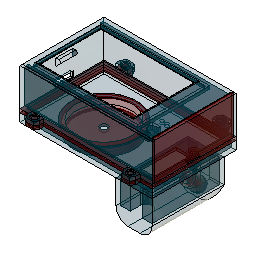
DicaPi v26 (Autodesk Fusion 360 design; units mm, degrees)
Autodesk Fusion 360 part; units mm, degrees
note: some values were not read from the file. Chosen so that the rebuilt part matches the saved one: which bodies a step acts on; which face or edge a step refers to. Set by a fixed rule: which sketch regions a step uses.
sketch "Mount-Grip" plane through (0, 0, 0) normal (0, 0, 1) x (1, 0, 0)
  line L0 (0, 0) -> (110, 0)
  line L1 (110, 0) -> (110, 70)
  line L2 (110, 70) -> (0, 70)
  line L3 (0, 70) -> (0, 0)
  circle A0 centre (35, 35) radius 25
  circle A1 centre (35, 35) radius 23
  line L4 (2, 68) -> (108, 68)
  line L5 (108, 68) -> (108, 2)
  line L6 (108, 2) -> (2, 2)
  line L7 (2, 2) -> (2, 68)
  circle A2 centre (60, 58.5) radius 1.5
  circle A3 centre (64, 58.5) radius 1.5
  line L8 (110, 60) -> (80, 60)
  line L9 (80, 60) -> (80, 0)
  line L10 (80, 0) -> (110, 0)
  line L11 (110, 0) -> (110, 60)
  circle A4 centre (95, 50) radius 2.5
  circle A5 centre (95, 10) radius 2.5
  line L12 (150, 60) -> (180, 60)
  line L13 (180, 60) -> (180, 0)
  line L14 (180, 0) -> (150, 0)
  line L15 (150, 0) -> (150, 60)
  line L16 (168, 51.7321) -> (165, 53.4641)
  line L17 (165, 53.4641) -> (162, 51.7321)
  line L18 (162, 51.7321) -> (162, 48.2679)
  line L19 (162, 48.2679) -> (165, 46.5359)
  line L20 (165, 46.5359) -> (168, 48.2679)
  line L21 (168, 48.2679) -> (168, 51.7321)
  line L22 (168, 11.7321) -> (165, 13.4641)
  line L23 (165, 13.4641) -> (162, 11.7321)
  line L24 (162, 11.7321) -> (162, 8.2679)
  line L25 (162, 8.2679) -> (165, 6.5359)
  line L26 (165, 6.5359) -> (168, 8.2679)
  line L27 (168, 8.2679) -> (168, 11.7321)
  circle A6 centre (35, 35) radius 27
  circle A7 centre (35, 35) radius 3
  circle A8 centre (165, 10) radius 2
  circle A9 centre (165, 50) radius 2
  line L28 (152, 15) -> (178, 15)
  line L29 (178, 15) -> (178, 45)
  line L30 (178, 45) -> (152, 45)
  line L31 (152, 45) -> (152, 15)
  line L32 (178, 15) -> (170, 15)
  line L33 (170, 15) -> (170, 2)
  line L34 (170, 2) -> (178, 2)
  line L35 (178, 2) -> (178, 15)
  line L36 (160, 15) -> (152, 15)
  line L37 (152, 15) -> (152, 2)
  line L38 (152, 2) -> (160, 2)
  line L39 (160, 2) -> (160, 15)
  line L40 (152, 45) -> (160, 45)
  line L41 (160, 45) -> (160, 58)
  line L42 (160, 58) -> (152, 58)
  line L43 (152, 58) -> (152, 45)
  line L44 (170, 58) -> (178, 58)
  line L45 (178, 58) -> (178, 45)
  line L46 (178, 45) -> (170, 45)
  line L47 (170, 45) -> (170, 58)
  line L48 (85, 15) -> (105, 15)
  line L49 (105, 15) -> (105, 45)
  line L50 (105, 45) -> (85, 45)
  line L51 (85, 45) -> (85, 15)
  point P0 (165, 50)
  point P1 (165, 10)
  dimension "d1" = 110
  dimension "d2" = 70
  dimension "d3" = 5
  dimension "d4" = 5
  dimension "d5" = 3
  dimension "d6" = 3
  dimension "d7" = 54
  dimension "d8" = 6
  dimension "d45" = 4
  dimension "d46" = 4
  constraint horizontal L0
  constraint vertical L1
  constraint horizontal L2
  constraint vertical L3
  constraint coincident L0.start L3.end
  constraint concentric A0 A1
  constraint horizontal L4
  constraint vertical L5
  constraint horizontal L6
  constraint vertical L7
  constraint horizontal L8
  constraint vertical L9
  constraint horizontal L10
  constraint vertical L11
  constraint coincident L0 L9.end
  constraint coincident L1 L8.start
  constraint horizontal L12
  constraint vertical L13
  constraint horizontal L14
  constraint vertical L15
  constraint concentric A1 A6
  constraint concentric A0 A7
  constraint coincident P1 A8.centre
  constraint coincident P0 A9.centre
  constraint horizontal L28
  constraint vertical L29
  constraint horizontal L30
  constraint vertical L31
  constraint horizontal L32
  constraint vertical L33
  constraint horizontal L34
  constraint vertical L35
  constraint horizontal L36
  constraint vertical L37
  constraint horizontal L38
  constraint vertical L39
  constraint coincident L28 L36.start
  constraint horizontal L40
  constraint vertical L41
  constraint horizontal L42
  constraint vertical L43
  constraint horizontal L44
  constraint vertical L45
  constraint horizontal L46
  constraint vertical L47
  constraint horizontal L48
  constraint vertical L49
  constraint horizontal L50
  constraint vertical L51
  measures "d1" distance of L0.start L0.end
  measures "d2" distance of L0.start L2.end
  measures "d3" diameter of A4
  measures "d4" diameter of A5
  measures "d5" distance of P0 L21
  measures "d6" distance of P1 L27
  measures "d7" diameter of A6
  measures "d8" diameter of A7
  measures "d45" diameter of A8
  measures "d46" diameter of A9
extrude "Extrude1" add sketch "Mount-Grip" along normal blind 2 contours L0 L1 L2 L3 L4 L5 L6 L7 L8 L9 | L0 L1 L5 L6 L8 L9 L10 L11 | L5 L6 L8 L9 | L4 L5 L6 L7 L8 L9 | A6 | L48 L49 L50 L51 makes body 1
extrude "Extrude2" add sketch "Mount-Grip" along normal blind 7 contours L0 L1 L2 L3 L4 L5 L6 L7 L8 L9 | L0 L1 L5 L6 L8 L9 L10 L11 bodies 1
chamfer "Chamfer1" distance 1 angle 45 1 edges at (92.6692, 50.904, 2) on bodies 1
chamfer "Chamfer2" distance 1 angle 45 1 edges at (92.6692, 10.904, 2) on bodies 1
extrude "Extrude3" add sketch "Mount-Grip" along normal blind 2 separate body contours A6 makes body 2
extrude "Extrude4" add sketch "Mount-Grip" along normal blind 2 contours A0 bodies 2
extrude "Extrude5" add sketch "Mount-Grip" against normal blind 2 contours A0 bodies 2
extrude "Extrude6" add sketch "Mount-Grip" along normal blind 2 contours A1 bodies 2
move_body "Move1" bodies 2 to x (1, 0, 0) y (0, 1, 0) z (0, 0, 1) at (0, 0, 2)
extrude "Extrude7" cut sketch "Mount-Grip" along normal blind 32 contours A1 bodies 2
extrude "Extrude8" add sketch "Mount-Grip" against normal blind 4 contours A0 bodies 2
extrude "Extrude9" add 1 faces at (59.2403, 33.758, -4) along direction (0, 0, -1) blind 2 on bodies 2 bodies 2
extrude "Extrude10" add sketch "Mount-Grip" against normal blind 4 contours A1 bodies 2
extrude "Extrude11" cut sketch "Mount-Grip" against normal blind 2 contours A1 bodies 2
extrude "Extrude12" cut sketch "Mount-Grip" along normal blind 4 contours A6 bodies 1
extrude "Extrude13" add sketch "Mount-Grip" along normal blind 1 contours A6 bodies 1
extrude "Extrude14" cut 1 faces at (60.4805, 32.516, 4) along direction (0, 0, -1) blind 1 on bodies 2 bodies 2
move_body "Move2" bodies 2 to x (1, 0, 0) y (0, 1, 0) z (0, 0, 1) at (0, 0, -1)
extrude "Extrude15" add sketch "Mount-Grip" along normal blind 30 separate body contours L12 L13 L14 L15 | L16 L17 L18 L19 L20 L21 | L22 L23 L24 L25 L26 L27 | A8 | A9 | L28 L29 L30 L31 L32 L36 L40 L46 | L28 L36 L37 L38 L39 | L30 L40 L41 L42 L43 | L28 L32 L33 L34 L35 | L30 L44 L45 L46 L47 makes body 3
chamfer "Chamfer3" distance 10 angle 45 1 edges at (165, 60, 30) on bodies 3
fillet "Fillet1" radius 10 2 edges at (180, 25, 30) (150, 25, 30) on bodies 3
extrude "Extrude16" cut sketch "Mount-Grip" along normal blind 3 contours L16 L17 L18 L19 L20 L21 | L22 L23 L24 L25 L26 L27 | A8 | A9 bodies 3
extrude "Extrude17" cut sketch "Mount-Grip" along normal blind 15 contours A8 | A9 bodies 3
extrude "Extrude18" cut sketch "Mount-Grip" along normal blind 20 contours L28 L29 L30 L31 L32 L36 L40 L46 | L28 L36 L37 L38 L39 | L30 L40 L41 L42 L43 | L28 L32 L33 L34 L35 | L30 L44 L45 L46 L47 bodies 3
fillet "Fillet2" radius 5 4 edges at (170, 15, 10) (160, 15, 10) (170, 45, 10) (160, 45, 10) on bodies 3
sketch "Button" plane through (0, 40, 40) normal (0, 0.707107, 0.707107) x (-1, 0, 0)
  ellipse E0 centre (-160, -28.2843) end of major axis (-160, -14.1421) minor radius 10 (-150, -28.2843) -> (-160, -14.1421) ccw
  line L0 (-160, -14.1421) -> (-170, -14.1421)
  ellipse E1 centre (-170, -28.2843) end of major axis (-170, -14.1421) minor radius 10 (-170, -14.1421) -> (-180, -28.2843) ccw
  line L1 (-180, -28.2843) -> (-150, -28.2843)
  line L2 (-161.5, -24.5) -> (-168.5, -24.5)
  line L3 (-168.5, -24.5) -> (-168.5, -17.5)
  line L4 (-168.5, -17.5) -> (-161.5, -17.5)
  line L5 (-161.5, -17.5) -> (-161.5, -24.5)
  line L6 (-161.5, -24.5) -> (-168.5, -17.5) construction
  line L7 (-168.5, -24.5) -> (-161.5, -17.5) construction
  circle A0 centre (-165, -21) radius 5
  circle A1 centre (-165, -21) radius 5.5
  circle A2 centre (-165, -21) radius 1.5
  point P0 (-165, -21)
  dimension "d52" = 7
  dimension "d53" = 7
  dimension "d68" = 3
  constraint horizontal L2
  constraint perpendicular L2 L3
  constraint parallel L2 L4
  constraint parallel L3 L5
  constraint coincident L6 P0
  constraint coincident L7 P0
  constraint coincident P0 A0.centre
  constraint concentric A0 A1
  constraint concentric A1 A2
  measures "d52" distance of L3.end L4.end
  measures "d53" distance of L2.end L3.end
  measures "d68" diameter of A2
extrude "Extrude19" cut sketch "Button" against normal blind 89 contours L2 L3 L4 L5 | A2 bodies 3
extrude "Extrude20" cut sketch "Button" against normal blind 43.5 contours A0 bodies 3
extrude "Extrude21" cut sketch "Button" against normal blind 57.5 contours A1 bodies 3
extrude "Extrude22" add sketch "Button" against normal blind 2 contours A1 bodies 3
extrude "Extrude23" add sketch "Button" against normal blind 1 separate body contours A1 makes body 4
extrude "Extrude24" add sketch "Button" against normal blind 1 contours L2 L3 L4 L5 | A0 | A2 bodies 4
extrude "Extrude25" add sketch "Button" along normal blind 3 contours L2 L3 L4 L5 | A0 | A2 bodies 4
extrude "Extrude26" cut sketch "Button" against normal blind 9 contours A2 bodies 4
move_body "Move3" bodies 4 to x (1, 0, 0) y (0, 1, 0) z (0, 0, 1) at (0, -2, -2)
move_body "Move4" bodies 4 to x (1, 0, 0) y (0, 1, 0) z (0, 0, 1) at (0, 0.5, 0.5)
fillet "Fillet3" radius 1 1 edges at (169.6616, 56.7491, 24.4936) on bodies 4
extrude "Extrude27" cut sketch "Mount-Grip" along normal blind 26 contours L48 L49 L50 L51 bodies 1
move_body "Move5" bodies 3 4 to x (-1, 0, 0) y (0, 1, 0) z (0, 0, -1) at (260, 0, 0)
extrude "Extrude28" add sketch "Button" against normal blind 10 separate body contours L2 L3 L4 L5 | A0 makes body 5
extrude "Extrude29" cut sketch "Button" against normal blind 4 contours L2 L3 L4 L5 bodies 5
move_face "OffsetFaces1" offset -2 1 faces at (164.7395, 48.1478, 20.5384) on bodies 5
extrude "Extrude30" add sketch "Button" against normal blind 10 contours A1 bodies 5
move_body "Move6" bodies 5 to x (-1, 0, 0) y (0, 1, 0) z (0, 0, -1) at (260, -2.88, 2.8812)
sketch "BodyBase" plane through (0, 0, 0) normal (0, 0, 1) x (1, 0, 0)
  line L0 (0, 0) -> (110, 0)
  line L1 (110, 0) -> (110, 70)
  line L2 (110, 70) -> (0, 70)
  line L3 (0, 70) -> (0, 0)
  line L4 (85, 35) -> (85, 60.5)
  line L5 (85, 60.5) -> (7, 60.5)
  line L6 (7, 60.5) -> (7, 35)
  line L7 (85, 35) -> (85, 9.5)
  line L8 (85, 9.5) -> (7, 9.5)
  line L9 (7, 9.5) -> (7, 35)
  line L10 (91, 35) -> (91, 63)
  line L11 (91, 63) -> (4, 63)
  line L12 (4, 63) -> (4, 35)
  line L13 (91, 35) -> (91, 7)
  line L14 (91, 7) -> (4, 7)
  line L15 (4, 7) -> (4, 35)
  line L16 (2, 68) -> (108, 68)
  line L17 (108, 68) -> (108, 2)
  line L18 (108, 2) -> (2, 2)
  line L19 (2, 2) -> (2, 68)
  line L20 (110, 68) -> (95, 68)
  line L21 (95, 68) -> (95, 2)
  line L22 (95, 2) -> (110, 2)
  line L23 (110, 2) -> (110, 68)
  line L24 (110, 68) -> (106, 68)
  line L25 (106, 68) -> (106, 2)
  line L26 (106, 2) -> (110, 2)
  line L27 (110, 2) -> (110, 68)
  line L28 (3, 67) -> (107, 67)
  line L29 (107, 67) -> (107, 3)
  line L30 (107, 3) -> (3, 3)
  line L31 (3, 3) -> (3, 67)
  dimension "d84" = 78
  dimension "d85" = 25.5
  dimension "d86" = 25.5
  dimension "d87" = 28
  constraint horizontal L0
  constraint vertical L1
  constraint horizontal L2
  constraint vertical L3
  constraint coincident L0.start L3.end
  constraint vertical L4
  constraint horizontal L5
  constraint vertical L6
  constraint vertical L7
  constraint horizontal L8
  constraint vertical L9
  constraint vertical L10
  constraint horizontal L11
  constraint vertical L12
  constraint vertical L13
  constraint horizontal L14
  constraint vertical L15
  constraint horizontal L16
  constraint vertical L17
  constraint horizontal L18
  constraint vertical L19
  constraint horizontal L20
  constraint vertical L21
  constraint horizontal L22
  constraint vertical L23
  constraint coincident L18 L21.end
  constraint coincident L1 L20.start
  constraint horizontal L24
  constraint vertical L25
  constraint horizontal L26
  constraint vertical L27
  constraint coincident L22 L25.end
  constraint horizontal L28
  constraint vertical L29
  constraint horizontal L30
  constraint vertical L31
  measures "d84" distance of L6.end L4.start
  measures "d85" distance of L6.end L5.end
  measures "d86" distance of L6.end L8.end
  measures "d87" distance of L12.end L14.end
extrude "Extrude31" add sketch "BodyBase" along normal blind 35 separate body contours L0 L1 L2 L3 L16 L18 L19 L20 L22 L24 L26 | L1 L17 L20 L22 L23 L24 L26 L27 | L16 L17 L18 L20 L22 L24 L25 L26 L28 L29 L30 | L18 L21 L22 L25 L30 | L16 L20 L21 L25 L28 | L16 L18 L19 L21 L28 L30 L31 | L21 L25 L28 L30 | L25 L28 L29 L30 | L21 L28 L30 L31 | L4 L5 L6 L7 L8 L9 | L10 L11 L12 L13 L14 L15 makes body 6
sketch "Face" plane through (0, 0, 35) normal (0, 0, 1) x (-1, 0, 0)
  line L0 (-110, 0) -> (-110, -70)
  line L1 (-110, -70) -> (0, -70)
  line L2 (0, -70) -> (0, 0)
  line L3 (0, 0) -> (-110, 0)
  line L4 (-95, -68) -> (-110, -68)
  line L5 (-110, -68) -> (-110, -2)
  line L6 (-110, -2) -> (-95, -2)
  line L7 (-95, -2) -> (-95, -68)
  line L8 (-108, -68) -> (-110, -68)
  line L9 (-110, -68) -> (-110, -2)
  line L10 (-110, -2) -> (-108, -2)
  line L11 (-108, -2) -> (-108, -68)
  line L12 (-108, -2) -> (-106, -2)
  line L13 (-106, -2) -> (-106, -68)
  line L14 (-106, -68) -> (-108, -68)
  line L15 (-108, -68) -> (-108, -2)
  line L16 (-7, -9.5) -> (-85, -9.5)
  line L17 (-85, -9.5) -> (-85, -60.5)
  line L18 (-85, -60.5) -> (-7, -60.5)
  line L19 (-7, -60.5) -> (-7, -9.5)
  line L20 (-4, -63) -> (-91, -63)
  line L21 (-91, -63) -> (-91, -7)
  line L22 (-91, -7) -> (-4, -7)
  line L23 (-4, -7) -> (-4, -63)
  line L24 (-2, -65) -> (-93, -65)
  line L25 (-93, -65) -> (-93, -5)
  line L26 (-93, -5) -> (-2, -5)
  line L27 (-2, -5) -> (-2, -65)
  constraint horizontal L4
  constraint vertical L5
  constraint horizontal L6
  constraint vertical L7
  constraint coincident L0 L5.end
  constraint horizontal L8
  constraint vertical L9
  constraint horizontal L10
  constraint vertical L11
  constraint coincident L4 L8.start
  constraint horizontal L12
  constraint vertical L13
  constraint horizontal L14
  constraint vertical L15
  constraint coincident L4 L13.end
  constraint horizontal L16
  constraint vertical L17
  constraint horizontal L18
  constraint vertical L19
  constraint horizontal L20
  constraint vertical L21
  constraint horizontal L22
  constraint vertical L23
  constraint horizontal L24
  constraint vertical L25
  constraint horizontal L26
  constraint vertical L27
sketch "Adhesive" plane through (0, 0, 0) normal (0, 0, -1) x (1, 0, 0)
  line L0 (110, -70) -> (110, 0)
  line L1 (110, 0) -> (0, 0)
  line L2 (0, 0) -> (0, -70)
  line L3 (0, -70) -> (110, -70)
  line L4 (2, -2) -> (106, -2)
  line L5 (106, -2) -> (106, -68)
  line L6 (106, -68) -> (2, -68)
  line L7 (2, -68) -> (2, -2)
  line L8 (108, -2) -> (110, -2)
  line L9 (110, -2) -> (110, -68)
  line L10 (110, -68) -> (108, -68)
  line L11 (108, -68) -> (108, -2)
  line L12 (3, -3) -> (107, -3)
  line L13 (107, -3) -> (107, -67)
  line L14 (107, -67) -> (3, -67)
  line L15 (3, -67) -> (3, -3)
  line L16 (108, -2) -> (106, -2)
  line L17 (106, -2) -> (106, -68)
  line L18 (106, -68) -> (108, -68)
  line L19 (108, -68) -> (108, -2)
  constraint horizontal L4
  constraint vertical L5
  constraint horizontal L6
  constraint vertical L7
  constraint horizontal L8
  constraint vertical L9
  constraint horizontal L10
  constraint vertical L11
  constraint coincident L0 L9.end
  constraint horizontal L12
  constraint vertical L13
  constraint horizontal L14
  constraint vertical L15
  constraint horizontal L16
  constraint vertical L17
  constraint horizontal L18
  constraint vertical L19
extrude "Extrude32" cut sketch "Adhesive" against normal blind 33.5 contours L5 L11 L12 L13 L14 L16 L17 L18 L19 | L4 L5 L6 L7 L12 L14 L15 L17 | L5 L12 L14 L15 L17 | L5 L12 L13 L14 L17 bodies 6
extrude "Extrude33" add sketch "Adhesive" against normal blind 2 contours L5 L11 L12 L13 L14 L16 L17 L18 L19 | L4 L5 L6 L7 L12 L14 L15 L17 bodies 6
extrude "Extrude34" add sketch "Adhesive" along normal blind 2 contours L5 L11 L12 L13 L14 L16 L17 L18 L19 | L4 L5 L6 L7 L12 L14 L15 L17 bodies 6
extrude "Extrude35" cut sketch "Face" against normal blind 5 contours L16 L17 L18 L19 bodies 6
extrude "Extrude36" add sketch "Face" against normal blind 4 contours L24 L25 L26 L27 bodies 6
extrude "Extrude37" cut sketch "Face" against normal blind 2 contours L0 L4 L5 L6 L8 L9 L10 L11 L15 | L4 L6 L11 L12 L13 L14 L15 | L4 L6 L7 L13 bodies 6
extrude "Extrude38" cut sketch "Face" against normal blind 30 contours L0 L4 L5 L6 L8 L9 L10 L11 L15 bodies 6
extrude "Extrude39" add sketch "Face" against normal blind 1.5 contours L4 L6 L7 L13 bodies 6
extrude "Extrude40" add 1 faces at (106, 24, 34.5) along direction (1, 0, 0) blind 2 on bodies 6 bodies 6
chamfer "Chamfer4" distance 1 angle 45 1 edges at (108, 35, 33.5) on bodies 6
sketch "IOCap" plane through (110, 0, 0) normal (1, 0, 0) x (0, 1, 0)
  line L0 (2, 5) -> (2, 35)
  line L1 (2, 35) -> (0, 35)
  line L2 (0, 35) -> (0, 0)
  line L3 (0, 0) -> (70, 0)
  line L4 (70, 0) -> (70, 35)
  line L5 (70, 35) -> (68, 35)
  line L6 (68, 35) -> (68, 5)
  line L7 (68, 5) -> (2, 5)
  line L8 (2, 35) -> (68, 35)
  line L9 (68, 35) -> (68, 3)
  line L10 (68, 3) -> (2, 3)
  line L11 (2, 3) -> (2, 35)
  line L12 (30, 3) -> (40, 3)
  line L13 (40, 3) -> (40, 4)
  line L14 (40, 4) -> (30, 4)
  line L15 (30, 4) -> (30, 3)
  line L16 (30, 3) -> (40, 3)
  line L17 (40, 3) -> (40, 5)
  line L18 (40, 5) -> (30, 5)
  line L19 (30, 5) -> (30, 3)
  constraint horizontal L8
  constraint vertical L9
  constraint horizontal L10
  constraint vertical L11
  constraint coincident L0.end L1.start
  constraint horizontal L12
  constraint vertical L13
  constraint horizontal L14
  constraint vertical L15
  constraint coincident L10 L12.start
  constraint horizontal L16
  constraint vertical L17
  constraint horizontal L18
  constraint vertical L19
  constraint coincident L7 L17.end
extrude "Extrude41" add 1 faces at (108, 46, 3) along direction (-1, 0, 0) blind 1 on bodies 6 bodies 6
extrude "Extrude42" cut sketch "IOCap" against normal blind 2 contours L7 L10 L11 L15 L19 | L7 L14 L17 L18 L19 | L7 L9 L10 L13 L17 | L10 L12 L13 L14 L15 L16 L17 L19 bodies 6
extrude "Extrude43" add sketch "IOCap" against normal blind 2 separate body contours L0 L6 L7 L8 L9 L11 L18 | L7 L10 L11 L15 L19 | L7 L9 L10 L13 L17 makes body 7
extrude "Extrude44" add sketch "IOCap" against normal blind 1 contours L7 L14 L17 L18 L19 bodies 7
sketch "Body-Top" plane through (0, 70, 0) normal (0, 1, 0) x (-1, 0, 0)
  line L0 (-110, 0) -> (0, 0)
  line L1 (0, 0) -> (0, 35)
  line L2 (0, 35) -> (-110, 35)
  line L3 (-110, 35) -> (-110, 0)
  line L4 (-100, 0) -> (-90, 0)
  line L5 (-90, 0) -> (-90, 5)
  line L6 (-90, 5) -> (-100, 5)
  line L7 (-100, 5) -> (-100, 0)
  line L8 (-10, 0) -> (-20, 0)
  line L9 (-20, 0) -> (-20, 5)
  line L10 (-20, 5) -> (-10, 5)
  line L11 (-10, 5) -> (-10, 0)
  line L12 (-20, 33) -> (-50, 33)
  line L13 (-50, 33) -> (-50, 18)
  line L14 (-50, 18) -> (-20, 18)
  line L15 (-20, 18) -> (-20, 33)
  line L16 (-23, 18) -> (-47, 18)
  line L17 (-47, 18) -> (-47, 33)
  line L18 (-47, 33) -> (-23, 33)
  line L19 (-23, 33) -> (-23, 18)
  constraint horizontal L4
  constraint vertical L5
  constraint horizontal L6
  constraint vertical L7
  constraint coincident L0 L4.start
  constraint horizontal L8
  constraint vertical L9
  constraint horizontal L10
  constraint vertical L11
  constraint coincident L0 L8.start
  constraint horizontal L12
  constraint vertical L13
  constraint horizontal L14
  constraint vertical L15
  constraint horizontal L16
  constraint vertical L17
  constraint horizontal L18
  constraint vertical L19
  constraint coincident L12 L17.end
  constraint coincident L14 L16.start
extrude "Extrude45" add sketch "Body-Top" along normal blind 15 separate body contours L12 L14 L16 L17 L18 L19 makes body 8
sketch "Body-Bottom" plane through (0, 0, 0) normal (0, -1, 0) x (1, 0, 0)
  line L0 (0, 0) -> (110, 0)
  line L1 (110, 0) -> (110, 35)
  line L2 (110, 35) -> (0, 35)
  line L3 (0, 35) -> (0, 0)
  line L4 (10, 0) -> (20, 0)
  line L5 (20, 0) -> (20, 5)
  line L6 (20, 5) -> (10, 5)
  line L7 (10, 5) -> (10, 0)
  line L8 (90, 0) -> (100, 0)
  line L9 (100, 0) -> (100, 5)
  line L10 (100, 5) -> (90, 5)
  line L11 (90, 5) -> (90, 0)
  constraint horizontal L4
  constraint vertical L5
  constraint horizontal L6
  constraint vertical L7
  constraint coincident L0 L4.start
  constraint horizontal L8
  constraint vertical L9
  constraint horizontal L10
  constraint vertical L11
  constraint coincident L0 L8.start
sketch "View-Guide" plane through (0, 0, 33) normal (0, 0, 1) x (-1, 0, 0)
  line L0 (-23, -70) -> (-47, -70)
  line L1 (-47, -70) -> (-47, -85)
  line L2 (-47, -85) -> (-23, -85)
  line L3 (-23, -85) -> (-23, -70)
  line L4 (-26, -83) -> (-44, -83)
  line L5 (-44, -83) -> (-44, -72)
  line L6 (-44, -72) -> (-26, -72)
  line L7 (-26, -72) -> (-26, -83)
  circle A0 centre (-35, -77.5) radius 5
  circle A1 centre (-35, -77.5) radius 4.75
  line L8 (-44, -77.25) -> (-26, -77.25)
  line L9 (-26, -77.25) -> (-26, -77.75)
  line L10 (-26, -77.75) -> (-44, -77.75)
  line L11 (-44, -77.75) -> (-44, -77.25)
  line L12 (-44, -77.25) -> (-26, -77.75) construction
  line L13 (-26, -77.25) -> (-44, -77.75) construction
  line L14 (-35.25, -72) -> (-34.75, -72)
  line L15 (-34.75, -72) -> (-34.75, -83)
  line L16 (-34.75, -83) -> (-35.25, -83)
  line L17 (-35.25, -83) -> (-35.25, -72)
  line L18 (-35.25, -72) -> (-34.75, -83) construction
  line L19 (-34.75, -72) -> (-35.25, -83) construction
  point P0 (-35, -77.5)
  point P1 (-35, -77.5)
  dimension "d119" = 18
  dimension "d120" = 11
  dimension "d123" = 9.5
  dimension "d124" = 0.5
  dimension "d125" = 0.5
  dimension "d126" = 11
  constraint horizontal L4
  constraint vertical L5
  constraint horizontal L6
  constraint vertical L7
  constraint concentric A0 A1
  constraint horizontal L8
  constraint perpendicular L8 L9
  constraint parallel L8 L10
  constraint parallel L9 L11
  constraint coincident L12 P1
  constraint coincident L13 P1
  constraint coincident P1 P0
  constraint horizontal L14
  constraint perpendicular L14 L15
  constraint parallel L14 L16
  constraint parallel L15 L17
  constraint coincident L18 P1
  constraint coincident L19 P1
  measures "d119" distance of L4.start L4.end
  measures "d120" distance of L4.start L6.end
  measures "d123" diameter of A1
  measures "d124" distance of L8.end L9.end
  measures "d125" distance of L15.end L16.end
  measures "d126" distance of L14.end L15.end
extrude "Extrude46" cut sketch "View-Guide" against normal blind 32 contours L4 L7 A0 L10 L15 | L4 A0 L15 L16 L17 | L7 A0 L8 L9 L10 | L4 L5 A0 L10 L17 | A0 A1 L10 L15 | A0 A1 L15 L17 | L6 L7 A0 L8 L15 | A0 A1 L8 L10 | A0 A1 L10 L17 | A1 L10 L15 | A1 L10 L15 L17 | A0 A1 L8 L15 | A1 L8 L10 L15 | L5 A0 L8 L10 L11 | A0 A1 L8 L10 | A1 L10 L17 | L8 L10 L15 L17 | L6 A0 L14 L15 L17 | A0 A1 L15 L17 | A1 L8 L15 | L5 L6 A0 L8 L17 | A0 A1 L8 L17 | A1 L8 L10 L17 | A1 L8 L15 L17 | A1 L8 L17 bodies 8
extrude "Extrude47" add sketch "View-Guide" against normal blind 0.5 contours L4 A0 L15 L16 L17 | L7 A0 L8 L9 L10 | A0 A1 L10 L15 | A0 A1 L15 L17 | A0 A1 L8 L10 | A0 A1 L10 L17 | A0 A1 L8 L15 | L5 A0 L8 L10 L11 | L6 A0 L14 L15 L17 | A0 A1 L15 L17 | A0 A1 L8 L17 picked at (-30.1719, -77.2778) bodies 8
extrude "Extrude48" add sketch "View-Guide" against normal blind 0.5 contours A0 A1 L8 L10 picked at (-39.8288, -77.6945) bodies 8
move_body "Move7" bodies 8 to x (-1, 0, 0) y (0, 1, 0) z (0, 0, -1) at (70, 0, 51)
extrude "Extrude49" add sketch "Body-Bottom" along normal blind 7 contours L0 L4 L5 L6 L7 | L0 L8 L9 L10 L11 bodies 6
extrude "Extrude50" add sketch "Body-Top" along normal blind 7 contours L0 L4 L5 L6 L7 | L0 L8 L9 L10 L11 bodies 6
chamfer "Chamfer5" distance 3 angle 45 8 edges at (10, 77, 2.5) (20, 77, 2.5) (90, 77, 2.5) (100, 77, 2.5) (10, -7, 2.5) (20, -7, 2.5) (100, -7, 2.5) (90, -7, 2.5) on bodies 6
sketch "Sketch14" plane through (0, 0, 0) normal (0, 0, -1) x (1, 0, 0)
  line L0 (93, 7) -> (90, 4)
  line L1 (90, 4) -> (90, 0)
  line L2 (90, 0) -> (20, 0)
  line L3 (20, 0) -> (20, 4)
  line L4 (20, 4) -> (17, 7)
  line L5 (17, 7) -> (13, 7)
  line L6 (13, 7) -> (10, 4)
  line L7 (10, 4) -> (10, 0)
  line L8 (10, 0) -> (0, 0)
  line L9 (0, 0) -> (0, -70)
  line L10 (0, -70) -> (10, -70)
  line L11 (10, -70) -> (10, -74)
  line L12 (10, -74) -> (13, -77)
  line L13 (13, -77) -> (17, -77)
  line L14 (17, -77) -> (20, -74)
  line L15 (20, -74) -> (20, -70)
  line L16 (20, -70) -> (90, -70)
  line L17 (90, -70) -> (90, -74)
  line L18 (90, -74) -> (93, -77)
  line L19 (93, -77) -> (97, -77)
  line L20 (97, -77) -> (100, -74)
  line L21 (100, -74) -> (100, -70)
  line L22 (100, -70) -> (110, -70)
  line L23 (110, -70) -> (110, 0)
  line L24 (110, 0) -> (100, 0)
  line L25 (100, 0) -> (100, 4)
  line L26 (100, 4) -> (97, 7)
  line L27 (97, 7) -> (93, 7)
  line L28 (2, -68) -> (2, -2)
  line L29 (2, -2) -> (108, -2)
  line L30 (108, -2) -> (108, -68)
  line L31 (108, -68) -> (2, -68)
  line L32 (13.2679, 6) -> (11.5359, 3)
  line L33 (11.5359, 3) -> (13.2679, 0)
  line L34 (13.2679, 0) -> (16.7321, 0)
  line L35 (16.7321, 0) -> (18.4641, 3)
  line L36 (18.4641, 3) -> (16.7321, 6)
  line L37 (16.7321, 6) -> (13.2679, 6)
  line L38 (93.268, 6) -> (91.5359, 3)
  line L39 (91.5359, 3) -> (93.268, 0)
  line L40 (93.268, 0) -> (96.7321, 0)
  line L41 (96.7321, 0) -> (98.4641, 3)
  line L42 (98.4641, 3) -> (96.7321, 6)
  line L43 (96.7321, 6) -> (93.268, 6)
  line L44 (13.2679, -70) -> (11.5359, -73)
  line L45 (11.5359, -73) -> (13.2679, -76)
  line L46 (13.2679, -76) -> (16.7321, -76)
  line L47 (16.7321, -76) -> (18.4641, -73)
  line L48 (18.4641, -73) -> (16.7321, -70)
  line L49 (16.7321, -70) -> (13.2679, -70)
  line L50 (93.268, -70) -> (91.5359, -73)
  line L51 (91.5359, -73) -> (93.268, -76)
  line L52 (93.268, -76) -> (96.7321, -76)
  line L53 (96.7321, -76) -> (98.4641, -73)
  line L54 (98.4641, -73) -> (96.7321, -70)
  line L55 (96.7321, -70) -> (93.268, -70)
  point P0 (15, 3)
  point P1 (95, 3)
  point P2 (15, -73)
  point P3 (95, -73)
delete_face "DeleteFace1" 1 faces at (98, -6, 1.6667) on bodies 6
delete_face "DeleteFace2" 1 faces at (12, -6, 3.3333) on bodies 6
delete_face "DeleteFace3" 1 faces at (92, -6, 3.3333) on bodies 6
delete_face "DeleteFace4" 1 faces at (19, -5, 1.6667) on bodies 6
delete_face "DeleteFace5" 1 faces at (98, 76, 3.3333) on bodies 6
delete_face "DeleteFace6" 1 faces at (91, 75, 1.6667) on bodies 6
delete_face "DeleteFace7" 1 faces at (19, 75, 1.6667) on bodies 6
delete_face "DeleteFace8" 1 faces at (12, 76, 3.3333) on bodies 6
chamfer "Chamfer6" distance 2 angle 60 8 edges at (10, -7, 2.5) (20, -7, 2.5) (90, -7, 2.5) (100, -7, 2.5) (20, 77, 2.5) (10, 77, 2.5) (90, 77, 2.5) (100, 77, 2.5) measured on face at (13.3333, -7, 1.6667) measured on face at (13.3333, -7, 1.6667) measured on face at (93.3333, -7, 1.6667) measured on face at (93.3333, -7, 1.6667) measured on face at (16.6667, 77, 1.6667) measured on face at (16.6667, 77, 1.6667) measured on face at (96.6667, 77, 1.6667) measured on face at (96.6667, 77, 1.6667) on bodies 6
extrude "Extrude51" add 1 faces at (37.3333, 67.6667, 2) along direction (0, 0, 1) blind 3 on bodies 6 bodies 6
extrude "Extrude52" add 4 faces at (94, -4.6906, 5) (16, -4.6906, 5) (16, 74.6906, 5) (94, 74.6906, 5) along direction (0, 0, 1) blind 1 on bodies 6 bodies 6
extrude "Extrude53" cut sketch "Sketch14" against normal blind 2 contours L32 L33 L34 L35 L36 L37 | L38 L39 L40 L41 L42 L43 | L44 L45 L46 L47 L48 L49 | L50 L51 L52 L53 L54 L55 bodies 6
sketch "Sketch15" plane through (0, 0, 6) normal (0, 0, 1) x (-1, 0, 0)
  line L0 (-100, -73.5359) -> (-98, -77)
  line L1 (-98, -77) -> (-92, -77)
  line L2 (-92, -77) -> (-90, -73.5359)
  line L3 (-90, -73.5359) -> (-90, -70)
  line L4 (-90, -70) -> (-100, -70)
  line L5 (-100, -70) -> (-100, -73.5359)
  circle A0 centre (-15, -73) radius 2
  circle A1 centre (-95, -73) radius 2
  circle A2 centre (-95, 3) radius 2
  circle A3 centre (-15, 3) radius 2
  circle A4 centre (-15, 3) radius 3
  circle A5 centre (-95, 3) radius 3
  circle A6 centre (-95, -73) radius 3
  circle A7 centre (-15, -73) radius 3
  constraint concentric A3 A4
  constraint concentric A2 A5
  constraint concentric A1 A6
  constraint concentric A0 A7
extrude "Extrude54" cut sketch "Sketch15" against normal blind 10 contours A0 | A1 | A2 | A3 bodies 6
extrude "Extrude55" cut sketch "Sketch15" against normal blind 1 contours A6 | A4 | A5 | A7 bodies 6
extrude "Extrude56" add 4 faces at (92.6673, 71.7107, 2) (15.0498, 75.6648, 2) (12.6673, -4.2893, 2) (97.3327, -4.2893, 2) along direction (0, 0, -1) blind 1 on bodies 6 bodies 6
split "Split1" by plane through (110, 40, 3) normal (0, 0, 1) bodies 6 makes body 9 at (100.3333, 43.5, 35)
sketch "Sketch17" plane through (0, 0, 0) normal (-1, 0, 0) x (0, -1, 0)
  line L0 (-70, 3) -> (0, 3)
  line L1 (0, 3) -> (0, 35)
  line L2 (0, 35) -> (-70, 35)
  line L3 (-70, 35) -> (-70, 3)
  line L4 (-35, 33.5) -> (-28, 33.5)
  line L5 (-28, 33.5) -> (-28, 9.5)
  line L6 (-28, 9.5) -> (-35, 9.5)
  line L7 (-35, 9.5) -> (-35, 33.5)
  line L8 (-35, 33.5) -> (-42, 33.5)
  line L9 (-42, 33.5) -> (-42, 9.5)
  line L10 (-42, 9.5) -> (-35, 9.5)
  line L11 (-35, 9.5) -> (-35, 33.5)
  line L12 (-42, 9.5) -> (-28, 9.5)
  line L13 (-28, 9.5) -> (-28, 5.5)
  line L14 (-28, 5.5) -> (-42, 5.5)
  line L15 (-42, 5.5) -> (-42, 9.5)
  line L16 (-5, 33.5) -> (-65, 33.5)
  line L17 (-65, 33.5) -> (-65, 26.5)
  line L18 (-65, 26.5) -> (-5, 26.5)
  line L19 (-5, 26.5) -> (-5, 33.5)
  line L20 (-65, 26.5) -> (-5, 26.5)
  line L21 (-5, 26.5) -> (-5, 25)
  line L22 (-5, 25) -> (-65, 25)
  line L23 (-65, 25) -> (-65, 26.5)
  line L24 (-42, 26.5) -> (-28, 26.5)
  line L25 (-28, 26.5) -> (-28, 21.5)
  line L26 (-28, 21.5) -> (-42, 21.5)
  line L27 (-42, 21.5) -> (-42, 26.5)
  dimension "d150" = 7
  dimension "d151" = 24
  dimension "d152" = 24
  dimension "d153" = 4
  dimension "d156" = 60
  dimension "d157" = 7
  constraint horizontal L4
  constraint vertical L5
  constraint horizontal L6
  constraint vertical L7
  constraint horizontal L8
  constraint vertical L9
  constraint horizontal L10
  constraint vertical L11
  constraint horizontal L12
  constraint vertical L13
  constraint horizontal L14
  constraint vertical L15
  constraint horizontal L16
  constraint vertical L17
  constraint horizontal L18
  constraint vertical L19
  constraint horizontal L20
  constraint vertical L21
  constraint horizontal L22
  constraint vertical L23
  constraint horizontal L24
  constraint vertical L25
  constraint horizontal L26
  constraint vertical L27
  constraint midpoint L5 L25.end
  constraint coincident L18 L24.start
  constraint coincident L9 L24.start
  measures "d150" distance of L4.start L4.end
  measures "d151" distance of L4.start L6.end
  measures "d152" distance of L4.start L6.end
  measures "d153" distance of L9.end L14.end
  measures "d156" distance of L16.start L16.end
  measures "d157" distance of L16.start L18.end
extrude "Extrude58" add sketch "Sketch17" against normal blind 7 contours L5 L7 L11 L18 L20 L22 L24 L25 | L7 L9 L11 L18 L20 L22 L24 L27 | L5 L7 L11 L22 L25 L26 | L7 L9 L11 L22 L26 L27 bodies 9
extrude "Extrude57" cut sketch "Sketch17" against normal blind 41 contours L6 L10 L12 L13 L14 L15 bodies 9
chamfer "Chamfer7" distance 4 angle 45 1 edges at (7, 35, 21.5) measured on face at (7, 37.3333, 24.8333) on bodies 9
fillet "Fillet4" radius 1 2 edges at (7, 35, 26.5) (7, 35, 25.5) on bodies 9
delete_face "DeleteFace9" 1 faces at (2.3333, 32.6667, 21.5) on bodies 9
chamfer "Chamfer8" distance 0.5 angle 45 4 edges at (2, 35, 9.5) (2, 28, 7.5) (2, 42, 7.5) (2, 35, 5.5) measured on face at (2, 11.6667, 18.8333) measured on face at (2, 11.6667, 18.8333) measured on face at (2, 11.6667, 18.8333) measured on face at (2, 11.6667, 18.8333) on bodies 9
chamfer "Chamfer9" distance 2 angle 25 4 edges at (46, 9.5, 35) (85, 35, 35) (7, 35, 35) (46, 60.5, 35) measured on face at (100.3333, 43.5, 35) measured on face at (100.3333, 43.5, 35) measured on face at (100.3333, 43.5, 35) measured on face at (100.3333, 43.5, 35) on bodies 9
move_body "Move8" bodies 8 6 9 7 to x (1, 0, 0) y (0, 1, 0) z (0, 0, 1) at (0, 0, 7)
fillet "Fillet5" radius 1 2 edges at (108, 35, 42) (110, 35, 42) on bodies 7
fillet "Fillet6" radius 2 2 edges at (108, 16, 10) (108, 54, 10) on bodies 7
sketch "Sketch18" plane through (0, 0, 40.5) normal (0, 0, -1) x (1, 0, 0)
  line L0 (107, -68) -> (107, -2)
  line L1 (107, -2) -> (2, -2)
  line L2 (2, -2) -> (2, -5)
  line L3 (2, -5) -> (93, -5)
  line L4 (93, -5) -> (93, -65)
  line L5 (93, -65) -> (2, -65)
  line L6 (2, -65) -> (2, -68)
  line L7 (2, -68) -> (107, -68)
  line L8 (103, -8.2679) -> (100, -6.5359)
  line L9 (100, -6.5359) -> (97, -8.2679)
  line L10 (97, -8.2679) -> (97, -11.7321)
  line L11 (97, -11.7321) -> (100, -13.4641)
  line L12 (100, -13.4641) -> (103, -11.7321)
  line L13 (103, -11.7321) -> (103, -8.2679)
  line L14 (100, -5) -> (95, -5)
  line L15 (95, -5) -> (95, -15)
  line L16 (95, -15) -> (100, -15)
  line L17 (100, -15) -> (100, -5)
  circle A0 centre (100, -10) radius 2
  point P0 (100, -10)
  constraint horizontal L14
  constraint vertical L15
  constraint horizontal L16
  constraint vertical L17
  constraint coincident P0 A0.centre
extrude "Extrude59" add sketch "Sketch18" along normal blind 6 contours L9 L10 L11 L17 A0 | L9 L10 L11 L14 L15 L16 L17 | L17 A0 picked at (99.3352, -9.9502) bodies 9
extrude "Extrude60" cut sketch "Sketch18" along normal blind 2.5 contours L8 L12 L13 L17 A0 | L9 L10 L11 L17 A0 | L17 A0 | L17 A0 bodies 9
extrude "Extrude61" cut sketch "Sketch18" along normal blind 7 contours L17 A0 | L17 A0 bodies 9
extrude "Extrude62" add 2 faces at (100, 6.512, 35.6667) (100, 13.488, 35.6667) along direction (1, 0, 0) blind 2 on bodies 9 bodies 9
delete_face "DeleteFace10" 1 faces at (6.5139, 37.3333, 32.1254) on bodies 9
fillet "Fillet7" radius 1.5 1 edges at (8, 35, 33.5) on bodies 9
chamfer "Chamfer10" distance 1 angle 45 8 edges at (55, 70, 42) (0, 35, 42) (110, 69, 42) (110, 1, 42) (55, 0, 42) (54.5, 68, 40.5) (2, 35, 38) (54.5, 2, 40.5) measured on face at (101, 25.8333, 42) measured on face at (101, 25.8333, 42) measured on face at (101, 25.8333, 42) measured on face at (101, 25.8333, 42) measured on face at (101, 25.8333, 42) measured on face at (72.3333, 68, 21.5) measured on face at (2, 11.6667, 25.8333) measured on face at (72.3333, 2, 21.5) on bodies 9
hidden bodies 8
equation "d84 = 83.000 mm - 5 mm"
equation "d85 = 27.500 mm - 2 mm"
equation "d86 = 27.500 mm - 2 mm"
named bodies: "Mount-Face", "Mount-Sensor", "Grip", "Button", "Button-Holder", "Body-Bracket", "IO-Cap", "ViewFinder", "Body"
